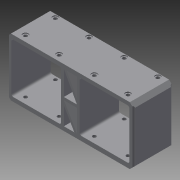
# Autodesk Inventor part: 2 cam holder 0.2 tolerance
Saved by Autodesk Inventor 2015 (Build 190159000, 159)
## iProperties
Created: 2015-03-12
Part Number: 2 cam holder 0.2 tolerance
Material: Nylon 6/6
Document SubType Name: Modeling
Designer: Vladimir
Density: 1.13 g/cm^3
Appearance: Nylon 6
Author: Vladimir
Autodesk Inventor part; units mm, degrees
ref_plane "YZ Plane" through (0, 0, 0) normal (1, 0, 0) x (0, 1, 0)
ref_plane "XZ Plane" through (0, 0, 0) normal (0, 1, 0) x (-1, 0, 0)
ref_plane "XY Plane" through (0, 0, 0) normal (0, 0, 1) x (1, 0, 0)
sketch "0.2mm tolerance" plane through (0, 0, 0) normal (0, 0, 1) x (1, 0, 0)
  line L0 (-41.2, -0.2479) -> (-41.2, 26.7521)
  line L1 (-13.4, -0.0479) -> (-38, -0.0479)
  line L2 (-39, 0.9521) -> (-39, 25.5521)
  line L3 (-38, 26.5521) -> (-13.4, 26.5521)
  line L4 (-12.4, 25.5521) -> (-12.4, 0.9521)
  line L5 (-1.4, 0.1521) -> (23.2, 0.1521)
  line L6 (24.2, 1.1521) -> (24.2, 25.7521)
  line L7 (23.2, 26.7521) -> (-1.4, 26.7521)
  line L8 (-2.4, 25.7521) -> (-2.4, 1.1521)
  line L9 (26.4, -0.2479) -> (26.4, 26.7521)
  line L10 (-39.2, -2.2479) -> (24.4, -2.2479)
  line L11 (-39.2, 28.7521) -> (24.4, 28.7521)
  line L12 (-10.9, 12.0286) -> (-3.9, -0.0479)
  line L13 (-5.287, -0.0479) -> (-10.9, 9.6357)
  line L14 (-5.287, -0.0479) -> (-10.9, -0.0479)
  line L15 (-3.9, -0.0479) -> (-3.9, 12.0286)
  line L16 (-10.9, 9.6357) -> (-10.9, -0.0479)
  line L17 (-10.9, 12.0286) -> (-3.9, 12.0286)
  arc A0 (-1.4, 26.7521) -> (-2.4, 25.7521) centre (-1.4, 25.7521) ccw
  arc A1 (-2.4, 1.1521) -> (-1.4, 0.1521) centre (-1.4, 1.1521) ccw
  arc A2 (23.2, 0.1521) -> (24.2, 1.1521) centre (23.2, 1.1521) ccw
  arc A3 (24.2, 25.7521) -> (23.2, 26.7521) centre (23.2, 25.7521) ccw
  arc A4 (-38, 26.5521) -> (-39, 25.5521) centre (-38, 25.5521) ccw
  arc A5 (-12.4, 25.5521) -> (-13.4, 26.5521) centre (-13.4, 25.5521) ccw
  arc A6 (-13.4, -0.0479) -> (-12.4, 0.9521) centre (-13.4, 0.9521) ccw
  arc A7 (-39, 0.9521) -> (-38, -0.0479) centre (-38, 0.9521) ccw
  line L18 (24.4, -2.2479) -> (26.4, -0.2479)
  line L19 (24.4, 28.7521) -> (26.4, 26.7521)
  line L20 (-41.2, -0.2479) -> (-39.2, -2.2479)
  line L21 (-39.2, 28.7521) -> (-41.2, 26.7521)
  line L22 (-3.9, 13.5286) -> (-10.9, 26.5521)
  line L23 (-9.5376, 26.5521) -> (-3.9, 16.0632)
  line L24 (-9.5376, 26.5521) -> (-3.9, 26.5521)
  line L25 (-10.9, 26.5521) -> (-10.9, 13.5286)
  line L26 (-3.9, 16.0632) -> (-3.9, 26.5521)
  line L27 (-3.9, 13.5286) -> (-10.9, 13.5286)
  point P0 (0, 0)
  point P1 (-41.2, 28.7521)
  point P2 (-41.2, -2.2479)
  point P3 (-12.4, -0.0479)
  point P4 (-39, 26.5521)
  point P5 (-39, -0.0479)
  point P6 (-12.4, 26.5521)
  point P7 (24.2, 26.7521)
  point P8 (-2.4, 26.7521)
  point P9 (26.4, 28.7521)
  point P10 (26.4, -2.2479)
  dimension "d11" = 31
  dimension "d12" = 26.6
  dimension "d13" = 26.6
  dimension "d14" = 26.6
  dimension "d46" = 2.2
  dimension "d47" = 2.2
  dimension "d48" = 67.6
  dimension "d68" = 1
  dimension "d69" = 1
  dimension "d70" = 1
  dimension "d71" = 1
  dimension "d72" = 1
  dimension "d73" = 1
  dimension "d74" = 1
  dimension "d75" = 1
  dimension "d76" = 2
  dimension "d77" = 2
  dimension "d78" = 2
  dimension "d79" = 2
  dimension "d80" = 2
  dimension "d81" = 2
  dimension "d82" = 2
  dimension "d83" = 2
  dimension "d253" = 26.6
  dimension "d254" = 1.5
  dimension "d255" = 1.2
  dimension "d263" = 2.2
  dimension "d267" = 2.2
  dimension "d268" = 2.2
  dimension "d273" = 1.5
  dimension "d277" = 10
  dimension "d279" = 2.2
  dimension "d280" = 2.2
  dimension "d281" = 2.2
  dimension "d282" = 1.5
  dimension "d283" = 1.2
  dimension "d284" = 1.5
  dimension "d285" = 1.5
  dimension "d286" = 1.5
  dimension "d287" = 1.5
  constraints: 56 end point, 20 point on line, 16 point on circle, 16 tangent, 8 centre point, 6 parallel, 6 perpendicular, 5 horizontal, 1 vertical
  measures "d11" distance of point (-41.2, -2.248) point (-41.2, 28.752)
  measures "d12" distance of point (-39, 26.552) point (-12.4, 26.552)
  measures "d13" distance of point (-39, -0.048) point (-39, 26.552)
  measures "d14" distance of point (-2.4, 26.752) point (24.2, 26.752)
  measures "d46" distance between parallel lines of L9 L6
  measures "d47" distance between parallel lines of L0 L2
  measures "d48" distance of point (-41.2, 28.752) point (26.4, 28.752)
  measures "d68" radius of A0
  measures "d69" radius of A1
  measures "d70" radius of A2
  measures "d71" radius of A3
  measures "d72" radius of A4
  measures "d73" radius of A5
  measures "d74" radius of A6
  measures "d75" radius of A7
  measures "d76" distance of L10.end point (26.4, -2.248)
  measures "d77" distance of L9.start point (26.4, -2.248)
  measures "d78" distance of L11.end point (26.4, 28.752)
  measures "d79" distance of L9.end point (26.4, 28.752)
  measures "d80" distance of L0.start point (-41.2, -2.248)
  measures "d81" distance of L10.start point (-41.2, -2.248)
  measures "d82" distance of L11.start point (-41.2, 28.752)
  measures "d83" distance of L0.end point (-41.2, 28.752)
  measures "d253" distance between parallel lines of L5 L7
  measures "d254" distance between parallel lines of L8 L15
  measures "d255" distance between parallel lines of L12 L13
  measures "d263" distance between parallel lines of L10 L14
  measures "d267" distance between parallel lines of L3 L11
  measures "d268" distance between parallel lines of L10 L1
  measures "d273" distance between parallel lines of L4 L16
  measures "d277" distance between parallel lines of L8 L4
  measures "d279" distance from line of L10 L12.end
  measures "d280" distance from line of L11 L25.start
  measures "d281" distance between parallel lines of L11 L24
  measures "d282" distance between parallel lines of L17 L27
  measures "d283" distance between parallel lines of L23 L22
  measures "d284" distance from line of L4 L12.start
  measures "d285" distance between parallel lines of L4 L25
  measures "d286" distance between parallel lines of L8 L26
  measures "d287" distance from line of L8 L22.start
extrude "Vol 0.2 mm" add sketch "0.2mm tolerance" along normal blind 21
sketch "0.2 mm mounting hole" plane through (-39.2, 28.7521, 0) normal (0, 1, 0) x (1, 0, 0)
  line L0 (-2, 0) -> (65.822, 0)
  line L1 (65.822, 0) -> (65.822, -21)
  line L2 (65.822, -21) -> (-2, -21)
  line L3 (-2, -21) -> (-2, 0)
  line L4 (0, -21) -> (63.6, -21) projected
  line L5 (-2, 0) -> (0.3, 0)
  line L6 (0.3, 0) -> (0.3, -21)
  line L7 (0.3, -21) -> (-2, -21)
  line L8 (-2, -21) -> (-2, 0)
  line L9 (0.3, 0) -> (26.7, 0)
  line L10 (26.7, 0) -> (26.7, -21)
  line L11 (26.7, -21) -> (0.3, -21)
  line L12 (0.3, -21) -> (0.3, 0)
  line L13 (65.822, -21) -> (63.522, -21)
  line L14 (63.522, -21) -> (63.522, 0)
  line L15 (63.522, 0) -> (65.822, 0)
  line L16 (65.822, 0) -> (65.822, -21)
  line L17 (0, 0) -> (63.6, 0) projected
  line L18 (63.522, -21) -> (37.122, -21)
  line L19 (37.122, -21) -> (37.122, 0)
  line L20 (37.122, 0) -> (63.522, 0)
  line L21 (63.522, 0) -> (63.522, -21)
  circle A0 centre (59.322, -1.7) radius 0.95
  circle A1 centre (41.322, -1.7) radius 0.95
  circle A2 centre (59.322, -17.7) radius 0.95
  circle A3 centre (41.322, -17.7) radius 0.95
  circle A4 centre (22.5, -1.7) radius 0.95
  circle A5 centre (4.5, -1.7) radius 0.95
  circle A6 centre (4.5, -17.7) radius 0.95
  circle A7 centre (22.5, -17.7) radius 0.95
  point P0 (39.2, 0)
  dimension "d296" = 2.3
  dimension "d297" = 26.4
  dimension "d298" = 2.3
  dimension "d299" = 26.4
  dimension "d300" = 1.9
  dimension "d301" = 1.9
  dimension "d302" = 18
  dimension "d303" = 4.2
  dimension "d304" = 4.2
  dimension "d305" = 1.7
  dimension "d306" = 1.9
  dimension "d307" = 1.9
  dimension "d308" = 16
  dimension "d309" = 16
  dimension "d310" = 1.9
  dimension "d311" = 1.9
  dimension "d312" = 1.9
  dimension "d313" = 1.9
  dimension "d314" = 16
  dimension "d315" = 1.7
  dimension "d316" = 1.7
  dimension "d317" = 18
  dimension "d318" = 4.2
  dimension "d319" = 4.2
  dimension "d320" = 4.2
  dimension "d321" = 4.2
  dimension "d322" = 16
  dimension "d323" = 18
  constraints: 40 end point, 10 parallel, 8 centre point, 5 horizontal, 5 perpendicular, 4 point on line
  measures "d296" distance of L6.end L7.end
  measures "d297" distance of L10.end L11.end
  measures "d298" distance of L14.end L15.end
  measures "d299" distance of L19.end L20.end
  measures "d300" diameter of A0
  measures "d301" diameter of A1
  measures "d302" distance of A1.centre A0.centre
  measures "d303" distance from line of A0.centre L21
  measures "d304" distance from line of L19 A1.centre
  measures "d305" distance from line of L20 A0.centre
  measures "d306" diameter of A2
  measures "d307" diameter of A3
  measures "d308" distance of A0.centre A2.centre
  measures "d309" distance of A1.centre A3.centre
  measures "d310" diameter of A4
  measures "d311" diameter of A5
  measures "d312" diameter of A6
  measures "d313" diameter of A7
  measures "d314" distance of A7.centre A4.centre
  measures "d315" distance from line of L9 A4.centre
  measures "d316" distance from line of L9 A5.centre
  measures "d317" distance of A4.centre A5.centre
  measures "d318" distance from line of L10 A4.centre
  measures "d319" distance from line of L6 A5.centre
  measures "d320" distance from line of L10 A7.centre
  measures "d321" distance from line of L6 A6.centre
  measures "d322" distance of A5.centre A6.centre
  measures "d323" distance of A6.centre A7.centre
hole "Hole 0.2mm" at (-41.2, 28.7521, 0) at (20.122, 28.7521, 1.7) at (20.122, 28.7521, 17.7) at (2.122, 28.7521, 17.7) at (2.122, 28.7521, 1.7) at (-16.7, 28.7521, 17.7) at (-16.7, 28.7521, 1.7) at (-34.7, 28.7521, 17.7) at (-34.7, 28.7521, 1.7) at (-41.2, 28.7521, 21) at (26.622, 28.7521, 21) at (26.622, 28.7521, 0) direction (0, -1, 0) diameter 1.9 end through all counterbore diameter 3 counterbore depth 0.5
body "Solid1"
